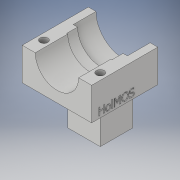
# Autodesk Inventor part: 5.1 Objektivhalterung_Unten
Saved by Autodesk Inventor 2018.3 (Build 223284000, 284)
## iProperties
Part Number: 5.1 Objektivhalterung_Unten
Material: Generisch
Document SubType Name: Modeling
Designer: pgmadmin
Density: 1 g/cm^3
Appearance: Vorgabe
Author: pgmadmin
Autodesk Inventor part; units mm, degrees
ref_plane "YZ Plane" through (0, 0, 0) normal (1, 0, 0) x (0, 1, 0)
ref_plane "XZ Plane" through (0, 0, 0) normal (0, 1, 0) x (-1, 0, 0)
ref_plane "XY Plane" through (0, 0, 0) normal (0, 0, 1) x (1, 0, 0)
sketch "Skizze1" plane through (0, 0, 0) normal (0, 0, 1) x (1, 0, 0)
  line L0 (-16, 20) -> (16, 20)
  line L1 (16, 20) -> (16, -20)
  line L2 (16, -20) -> (-16, -20)
  line L3 (-16, -20) -> (-16, 20)
  line L4 (-16, 20) -> (16, -20) construction
  line L5 (16, 20) -> (-16, -20) construction
  point P0 (0, 0)
  dimension "d0" = 32
  dimension "d1" = 40
  constraints: 12 end point, 2 midpoint, 2 parallel, 1 horizontal, 1 perpendicular
  measures "d0" distance of L1.end L2.end
  measures "d1" distance of L0.end L1.end
extrude "Extrusion1" add sketch "Skizze1" along normal blind 15
sketch "Skizze2" plane through (-16, -20, 0) normal (0, -1, 0) x (1, 0, 0)
  line L0 (0, 15) -> (32, 15) projected
  line L1 (0, 0) -> (0, 15) projected
  line L2 (32, 0) -> (0, 0) projected
  line L3 (32, 0) -> (32, 15) projected
  line L4 (32, 15) -> (0, 15) projected
  circle A0 centre (16, 15) radius 10
  point P0 (16, 0)
  dimension "d4" = 20
  constraints: 1 centre point, 1 midpoint
  measures "d4" diameter of A0
extrude "Extrusion2" cut sketch "Skizze2" against normal blind 15 contours A0 L0 | L0 A0
sketch "Skizze3" plane through (-16, -5, 0) normal (0, -1, 0) x (1, 0, 0)
  line L0 (0, 0) -> (0, 15) projected
  line L1 (32, 0) -> (0, 0) projected
  line L2 (32, 0) -> (32, 15) projected
  line L3 (26, 15) -> (32, 15) projected
  line L4 (0, 15) -> (6, 15) projected
  line L5 (6, 15) -> (26, 15) projected
  circle A0 centre (16, 15) radius 10.5
  point P0 (16, 0)
  dimension "d7" = 21
  constraints: 1 centre point, 1 midpoint
  measures "d7" diameter of A0
extrude "Extrusion3" cut sketch "Skizze3" against normal blind 5 contours A0 L3 L5 L4 | L4 L5 L3 A0
sketch "Skizze4" plane through (-16, 0, 0) normal (0, -1, 0) x (1, 0, 0)
  line L0 (5.5, 15) -> (26.5, 15) projected
  circle A0 centre (16, 15) radius 12.5
  point P0 (16, 0)
  dimension "d10" = 25
  constraints: 1 centre point, 1 midpoint
  measures "d10" diameter of A0
extrude "Extrusion4" cut sketch "Skizze4" against normal through all
sketch "Skizze5" plane through (0, 0, 15) normal (0, 0, 1) x (1, 0, 0)
  line L0 (-16, 20) -> (-16, -20) projected
  line L1 (-16, -20) -> (-10, -20) projected
  line L2 (-10, -20) -> (-10, -5) projected
  line L3 (10, -5) -> (10, -20) projected
  line L4 (10, -20) -> (16, -20) projected
  line L5 (16, -20) -> (16, 20) projected
  circle A0 centre (-13, -13) radius 1.8
  circle A1 centre (13, -13) radius 1.8
  point P0 (0, 0)
  dimension "d13" = 3.6
  dimension "d14" = 3.6
  dimension "d15" = 7
  dimension "d16" = 7
  dimension "d17" = 3
  dimension "d18" = 3
  constraints: 2 centre point
  measures "d13" diameter of A0
  measures "d14" diameter of A1
  measures "d15" distance from line of L1 A0.centre
  measures "d16" distance from line of L4 A1.centre
  measures "d17" distance from line of L5 A1.centre
  measures "d18" distance from line of L0 A0.centre
extrude "Extrusion5" cut sketch "Skizze5" against normal through all
sketch "Skizze6" plane through (0, 0, 0) normal (0, 0, -1) x (-1, 0, 0)
  line L0 (-7.5, 7.5) -> (7.5, 7.5)
  line L1 (7.5, 7.5) -> (7.5, -7.5)
  line L2 (7.5, -7.5) -> (-7.5, -7.5)
  line L3 (-7.5, -7.5) -> (-7.5, 7.5)
  line L4 (-7.5, 7.5) -> (7.5, -7.5) construction
  line L5 (7.5, 7.5) -> (-7.5, -7.5) construction
  point P0 (0, 0)
  dimension "d21" = 15
  dimension "d22" = 15
  constraints: 12 end point, 2 midpoint, 2 parallel, 1 horizontal, 1 perpendicular
  measures "d21" distance of L1.end L2.end
  measures "d22" distance of L0.end L1.end
extrude "Extrusion6" add sketch "Skizze6" along normal blind 20
sketch "Skizze7" plane through (0, 0, -20) normal (0, 0, -1) x (-1, 0, 0)
  circle A0 centre (0, 0) radius 2.5
  dimension "d25" = 5
  constraints: 1 centre point, 1 coincident
  measures "d25" diameter of A0
extrude "Extrusion7" cut sketch "Skizze7" against normal blind 7
sketch "Skizze8" plane through (0, 0, 0) normal (0, 0, -1) x (-1, 0, 0)
  line L0 (12.5, 20) -> (16, 20) projected
  line L1 (16, 20) -> (16, 10.5)
  line L2 (16, 20) -> (16, -20) projected
  line L3 (16, 10.5) -> (-16, 10.5)
  line L4 (-16, 20) -> (-16, -20) projected
  line L5 (16, 20) -> (-16, 20) projected
  line L6 (-16, 20) -> (16, 20)
  point P0 (0, 0)
  dimension "d28" = 9.5
  constraints: 6 end point, 2 point on line, 1 collinear, 1 perpendicular
  measures "d28" distance of L0.end L1.end
extrude "Extrusion8" cut sketch "Skizze8" along normal mid plane 58.75
sketch "Skizze9" plane through (16, -20, 15) normal (1, 0, 0) x (0, 0, -1)
  line L0 (15, 0) -> (0, 0) projected
  line L1 (14, 0) -> (14, 30.5)
  line L2 (0, 30.5) -> (15, 30.5) projected
  line L3 (15, 30.5) -> (15, 0) projected
  line L4 (14, 5.9024) -> (14, 5.4372)
  line L5 (14, 5.4372) -> (12.2869, 5.4372)
  line L6 (12.2869, 5.4372) -> (12.2869, 3.8262)
  line L7 (12.2869, 3.8262) -> (14, 3.8262)
  line L8 (14, 3.8262) -> (14, 3.361)
  line L9 (14, 3.361) -> (10.5, 3.361)
  line L10 (10.5, 3.361) -> (10.5, 3.8262)
  line L11 (10.5, 3.8262) -> (11.8728, 3.8262)
  line L12 (11.8728, 3.8262) -> (11.8728, 5.4372)
  line L13 (11.8728, 5.4372) -> (10.5, 5.4372)
  line L14 (10.5, 5.4372) -> (10.5, 5.9024)
  line L15 (10.5, 5.9024) -> (14, 5.9024)
  spline S0 degree 2 poles (12.6868, 8.7358) (13.3505, 8.7358) (14.0737, 8.0976) (14.0737, 7.5644) knots 0 0 0 1 2 2 2
  spline S1 degree 2 poles (14.0737, 7.5644) (14.0737, 7.017) (13.3278, 6.3902) (12.6868, 6.3902) knots 0 0 0 1 2 2 2
  spline S2 degree 2 poles (12.6868, 6.3902) (12.0288, 6.3902) (11.2998, 7.0369) (11.2998, 7.5644) knots 0 0 0 1 2 2 2
  spline S3 degree 2 poles (11.2998, 7.5644) (11.2998, 8.0976) (12.0259, 8.7358) (12.6868, 8.7358) knots 0 0 0 1 2 2 2
  spline S4 degree 2 poles (12.6868, 8.2792) (12.1763, 8.2792) (11.6799, 7.9076) (11.6799, 7.5644) knots 0 0 0 1 2 2 2
  spline S5 degree 2 poles (11.6799, 7.5644) (11.6799, 7.2212) (12.1763, 6.8468) (12.6868, 6.8468) knots 0 0 0 1 2 2 2
  spline S6 degree 2 poles (12.6868, 6.8468) (13.1831, 6.8468) (13.6937, 7.2212) (13.6937, 7.5644) knots 0 0 0 1 2 2 2
  spline S7 degree 2 poles (13.6937, 7.5644) (13.6937, 7.9048) (13.1917, 8.2792) (12.6868, 8.2792) knots 0 0 0 1 2 2 2
  line L16 (14, 9.6406) -> (14, 9.1981)
  line L17 (14, 9.1981) -> (10.344, 9.1981)
  line L18 (10.344, 9.1981) -> (10.344, 9.6406)
  line L19 (10.344, 9.6406) -> (14, 9.6406)
  line L20 (14, 13.325) -> (14, 12.8598)
  line L21 (14, 12.8598) -> (10.985, 12.8598)
  line L22 (10.985, 12.8598) -> (13.0357, 11.9465)
  line L23 (13.0357, 11.9465) -> (13.0357, 11.6629)
  line L24 (13.0357, 11.6629) -> (10.985, 10.7581)
  line L25 (10.985, 10.7581) -> (14, 10.7581)
  line L26 (14, 10.7581) -> (14, 10.3241)
  line L27 (14, 10.3241) -> (10.5, 10.3241)
  line L28 (10.5, 10.3241) -> (10.5, 10.9595)
  line L29 (10.5, 10.9595) -> (12.4485, 11.8331)
  line L30 (12.4485, 11.8331) -> (10.5, 12.6783)
  line L31 (10.5, 12.6783) -> (10.5, 13.325)
  line L32 (10.5, 13.325) -> (14, 13.325)
  spline S8 degree 2 poles (10.8999, 16.5101) (11.1325, 16.7087) (11.8132, 16.9299) (12.25, 16.9299) knots 0 0 0 1 2 2 2
  spline S9 degree 2 poles (12.25, 16.9299) (12.6754, 16.9299) (13.3647, 16.7143) (13.5972, 16.5101) knots 0 0 0 1 2 2 2
  spline S10 degree 2 poles (13.5972, 16.5101) (13.8412, 16.2946) (14.0737, 15.7245) (14.0737, 15.3813) knots 0 0 0 1 2 2 2
  spline S11 degree 2 poles (14.0737, 15.3813) (14.0737, 15.0267) (13.8327, 14.4595) (13.5972, 14.2524) knots 0 0 0 1 2 2 2
  spline S12 degree 2 poles (13.5972, 14.2524) (13.3647, 14.0511) (12.6811, 13.8355) (12.25, 13.8355) knots 0 0 0 1 2 2 2
  spline S13 degree 2 poles (12.25, 13.8355) (11.8104, 13.8355) (11.141, 14.0539) (10.8999, 14.2553) knots 0 0 0 1 2 2 2
  spline S14 degree 2 poles (10.8999, 14.2553) (10.6673, 14.4595) (10.4263, 15.0296) (10.4263, 15.3813) knots 0 0 0 1 2 2 2
  spline S15 degree 2 poles (10.4263, 15.3813) (10.4263, 15.7387) (10.6759, 16.3116) (10.8999, 16.5101) knots 0 0 0 1 2 2 2
  spline S16 degree 2 poles (12.25, 16.4449) (11.904, 16.4449) (11.3679, 16.2946) (11.1921, 16.1584) knots 0 0 0 1 2 2 2
  spline S17 degree 2 poles (11.1921, 16.1584) (11.0105, 16.0194) (10.829, 15.628) (10.829, 15.3841) knots 0 0 0 1 2 2 2
  spline S18 degree 2 poles (10.829, 15.3841) (10.829, 15.1317) (11.0049, 14.7516) (11.1921, 14.607) knots 0 0 0 1 2 2 2
  spline S19 degree 2 poles (11.1921, 14.607) (11.3707, 14.468) (11.9096, 14.3205) (12.25, 14.3205) knots 0 0 0 1 2 2 2
  spline S20 degree 2 poles (12.25, 14.3205) (12.9392, 14.3205) (13.671, 14.8991) (13.671, 15.3841) knots 0 0 0 1 2 2 2
  spline S21 degree 2 poles (13.671, 15.3841) (13.671, 15.8691) (12.9392, 16.4449) (12.25, 16.4449) knots 0 0 0 1 2 2 2
  spline S22 degree 2 poles (14.0624, 18.4161) (14.0624, 18.0361) (13.9036, 17.5028) (13.7901, 17.2674) knots 0 0 0 1 2 2 2
  line L33 (13.7901, 17.2674) -> (13.2058, 17.2674)
  line L34 (13.2058, 17.2674) -> (13.2058, 17.3015)
  spline S23 degree 2 poles (13.2058, 17.3015) (13.4214, 17.5312) (13.6596, 18.1126) (13.6596, 18.3821) knots 0 0 0 1 2 2 2
  spline S24 degree 2 poles (13.6596, 18.3821) (13.6596, 18.7678) (13.3391, 19.1621) (13.0754, 19.1621) knots 0 0 0 1 2 2 2
  spline S25 degree 2 poles (13.0754, 19.1621) (12.8655, 19.1621) (12.6045, 18.955) (12.5393, 18.731) knots 0 0 0 1 2 2 2
  spline S26 degree 2 poles (12.5393, 18.731) (12.4939, 18.5693) (12.4315, 18.2998) (12.3805, 18.0985) knots 0 0 0 1 2 2 2
  spline S27 degree 2 poles (12.3805, 18.0985) (12.3323, 17.9169) (12.1876, 17.6305) (12.0713, 17.5199) knots 0 0 0 1 2 2 2
  spline S28 degree 2 poles (12.0713, 17.5199) (11.955, 17.4121) (11.643, 17.293) (11.4388, 17.293) knots 0 0 0 1 2 2 2
  spline S29 degree 2 poles (11.4388, 17.293) (11.0134, 17.293) (10.4376, 17.9566) (10.4376, 18.47) knots 0 0 0 1 2 2 2
  spline S30 degree 2 poles (10.4376, 18.47) (10.4376, 18.765) (10.5539, 19.2869) (10.6645, 19.5109) knots 0 0 0 1 2 2 2
  line L35 (10.6645, 19.5109) -> (11.2204, 19.5109)
  line L36 (11.2204, 19.5109) -> (11.2204, 19.4769)
  spline S31 degree 2 poles (11.2204, 19.4769) (11.0673, 19.3096) (10.8404, 18.7877) (10.8404, 18.5012) knots 0 0 0 1 2 2 2
  spline S32 degree 2 poles (10.8404, 18.5012) (10.8404, 18.1779) (11.1438, 17.778) (11.3906, 17.778) knots 0 0 0 1 2 2 2
  spline S33 degree 2 poles (11.3906, 17.778) (11.6118, 17.778) (11.8756, 18.0134) (11.9352, 18.2346) knots 0 0 0 1 2 2 2
  spline S34 degree 2 poles (11.9352, 18.2346) (11.9749, 18.3821) (12.077, 18.8104) (12.1195, 18.9522) knots 0 0 0 1 2 2 2
  spline S35 degree 2 poles (12.1195, 18.9522) (12.2301, 19.3124) (12.6754, 19.6471) (13.0016, 19.6471) knots 0 0 0 1 2 2 2
  spline S36 degree 2 poles (13.0016, 19.6471) (13.2087, 19.6471) (13.6058, 19.4797) (13.7447, 19.3294) knots 0 0 0 1 2 2 2
  spline S37 degree 2 poles (13.7447, 19.3294) (13.8979, 19.1621) (14.0624, 18.7366) (14.0624, 18.4161) knots 0 0 0 1 2 2 2
  point P0 (15, 20)
  dimension "d31" = 1
  constraints: 2 end point, 2 point on line, 2 vertical
  measures "d31" distance between parallel lines of L1 L3
extrude "Extrusion9" cut sketch "Skizze9" against normal blind 2 contours L9 L10 L11 L12 L13 L14 L15 L1 L5 L6 L7 | S37 S22 L1 | L1 S22 L33 L34 S23 S24 S25 S26 S27 S28 S29 S30 L35 L36 S31 S32 S33 S34 S35 S36 S37 | S10 S11 L1 | L1 S11 S12 S13 S14 S15 S8 S9 S10 | S1 S2 S3 S0 L1 | L1 S0 S1 | L1 L21 L22 L23 L24 L25 L27 L28 L29 L30 L31 L32 | L17 L18 L19 L1
sketch "Skizze10" plane through (-16, -20, 0) normal (-1, 0, 0) x (0, 0, 1)
  line L0 (1, 30.5408) -> (1, 0)
  line L1 (0, 0) -> (15, 0) projected
  line L2 (0, 0) -> (0, 30.5) projected
  line L3 (1, 15.3671) -> (1, 15.8323)
  line L4 (1, 15.8323) -> (2.7131, 15.8323)
  line L5 (2.7131, 15.8323) -> (2.7131, 17.4433)
  line L6 (2.7131, 17.4433) -> (1, 17.4433)
  line L7 (1, 17.4433) -> (1, 17.9084)
  line L8 (1, 17.9084) -> (4.5, 17.9084)
  line L9 (4.5, 17.9084) -> (4.5, 17.4433)
  line L10 (4.5, 17.4433) -> (3.1272, 17.4433)
  line L11 (3.1272, 17.4433) -> (3.1272, 15.8323)
  line L12 (3.1272, 15.8323) -> (4.5, 15.8323)
  line L13 (4.5, 15.8323) -> (4.5, 15.3671)
  line L14 (4.5, 15.3671) -> (1, 15.3671)
  spline S0 degree 2 poles (2.3132, 12.5336) (1.6495, 12.5336) (0.9263, 13.1718) (0.9263, 13.705) knots 0 0 0 1 2 2 2
  spline S1 degree 2 poles (0.9263, 13.705) (0.9263, 14.2524) (1.6722, 14.8793) (2.3132, 14.8793) knots 0 0 0 1 2 2 2
  spline S2 degree 2 poles (2.3132, 14.8793) (2.9712, 14.8793) (3.7002, 14.2326) (3.7002, 13.705) knots 0 0 0 1 2 2 2
  spline S3 degree 2 poles (3.7002, 13.705) (3.7002, 13.1718) (2.9741, 12.5336) (2.3132, 12.5336) knots 0 0 0 1 2 2 2
  spline S4 degree 2 poles (2.3132, 12.9903) (2.8237, 12.9903) (3.3201, 13.3618) (3.3201, 13.705) knots 0 0 0 1 2 2 2
  spline S5 degree 2 poles (3.3201, 13.705) (3.3201, 14.0482) (2.8237, 14.4226) (2.3132, 14.4226) knots 0 0 0 1 2 2 2
  spline S6 degree 2 poles (2.3132, 14.4226) (1.8169, 14.4226) (1.3063, 14.0482) (1.3063, 13.705) knots 0 0 0 1 2 2 2
  spline S7 degree 2 poles (1.3063, 13.705) (1.3063, 13.3647) (1.8083, 12.9903) (2.3132, 12.9903) knots 0 0 0 1 2 2 2
  line L15 (1, 11.6289) -> (1, 12.0713)
  line L16 (1, 12.0713) -> (4.656, 12.0713)
  line L17 (4.656, 12.0713) -> (4.656, 11.6289)
  line L18 (4.656, 11.6289) -> (1, 11.6289)
  line L19 (1, 7.9445) -> (1, 8.4096)
  line L20 (1, 8.4096) -> (4.015, 8.4096)
  line L21 (4.015, 8.4096) -> (1.9643, 9.3229)
  line L22 (1.9643, 9.3229) -> (1.9643, 9.6066)
  line L23 (1.9643, 9.6066) -> (4.015, 10.5113)
  line L24 (4.015, 10.5113) -> (1, 10.5113)
  line L25 (1, 10.5113) -> (1, 10.9453)
  line L26 (1, 10.9453) -> (4.5, 10.9453)
  line L27 (4.5, 10.9453) -> (4.5, 10.31)
  line L28 (4.5, 10.31) -> (2.5515, 9.4364)
  line L29 (2.5515, 9.4364) -> (4.5, 8.5912)
  line L30 (4.5, 8.5912) -> (4.5, 7.9445)
  line L31 (4.5, 7.9445) -> (1, 7.9445)
  spline S8 degree 2 poles (4.1001, 4.7593) (3.8675, 4.5608) (3.1868, 4.3395) (2.75, 4.3395) knots 0 0 0 1 2 2 2
  spline S9 degree 2 poles (2.75, 4.3395) (2.3246, 4.3395) (1.6353, 4.5551) (1.4028, 4.7593) knots 0 0 0 1 2 2 2
  spline S10 degree 2 poles (1.4028, 4.7593) (1.1588, 4.9749) (0.9263, 5.545) (0.9263, 5.8882) knots 0 0 0 1 2 2 2
  spline S11 degree 2 poles (0.9263, 5.8882) (0.9263, 6.2427) (1.1673, 6.81) (1.4028, 7.017) knots 0 0 0 1 2 2 2
  spline S12 degree 2 poles (1.4028, 7.017) (1.6353, 7.2184) (2.3189, 7.434) (2.75, 7.434) knots 0 0 0 1 2 2 2
  spline S13 degree 2 poles (2.75, 7.434) (3.1896, 7.434) (3.859, 7.2156) (4.1001, 7.0142) knots 0 0 0 1 2 2 2
  spline S14 degree 2 poles (4.1001, 7.0142) (4.3327, 6.81) (4.5737, 6.2399) (4.5737, 5.8882) knots 0 0 0 1 2 2 2
  spline S15 degree 2 poles (4.5737, 5.8882) (4.5737, 5.5308) (4.3241, 4.9579) (4.1001, 4.7593) knots 0 0 0 1 2 2 2
  spline S16 degree 2 poles (2.75, 4.8246) (3.096, 4.8246) (3.6321, 4.9749) (3.8079, 5.111) knots 0 0 0 1 2 2 2
  spline S17 degree 2 poles (3.8079, 5.111) (3.9895, 5.25) (4.171, 5.6414) (4.171, 5.8853) knots 0 0 0 1 2 2 2
  spline S18 degree 2 poles (4.171, 5.8853) (4.171, 6.1378) (3.9951, 6.5178) (3.8079, 6.6625) knots 0 0 0 1 2 2 2
  spline S19 degree 2 poles (3.8079, 6.6625) (3.6293, 6.8015) (3.0904, 6.9489) (2.75, 6.9489) knots 0 0 0 1 2 2 2
  spline S20 degree 2 poles (2.75, 6.9489) (2.0608, 6.9489) (1.329, 6.3703) (1.329, 5.8853) knots 0 0 0 1 2 2 2
  spline S21 degree 2 poles (1.329, 5.8853) (1.329, 5.4003) (2.0608, 4.8246) (2.75, 4.8246) knots 0 0 0 1 2 2 2
  spline S22 degree 2 poles (0.9376, 2.8533) (0.9376, 3.2334) (1.0964, 3.7666) (1.2099, 4.002) knots 0 0 0 1 2 2 2
  line L32 (1.2099, 4.002) -> (1.7942, 4.002)
  line L33 (1.7942, 4.002) -> (1.7942, 3.968)
  spline S23 degree 2 poles (1.7942, 3.968) (1.5786, 3.7383) (1.3404, 3.1568) (1.3404, 2.8874) knots 0 0 0 1 2 2 2
  spline S24 degree 2 poles (1.3404, 2.8874) (1.3404, 2.5016) (1.6609, 2.1074) (1.9246, 2.1074) knots 0 0 0 1 2 2 2
  spline S25 degree 2 poles (1.9246, 2.1074) (2.1345, 2.1074) (2.3955, 2.3144) (2.4607, 2.5385) knots 0 0 0 1 2 2 2
  spline S26 degree 2 poles (2.4607, 2.5385) (2.5061, 2.7002) (2.5685, 2.9696) (2.6195, 3.171) knots 0 0 0 1 2 2 2
  spline S27 degree 2 poles (2.6195, 3.171) (2.6677, 3.3525) (2.8124, 3.639) (2.9287, 3.7496) knots 0 0 0 1 2 2 2
  spline S28 degree 2 poles (2.9287, 3.7496) (3.045, 3.8574) (3.357, 3.9765) (3.5612, 3.9765) knots 0 0 0 1 2 2 2
  spline S29 degree 2 poles (3.5612, 3.9765) (3.9866, 3.9765) (4.5624, 3.3128) (4.5624, 2.7994) knots 0 0 0 1 2 2 2
  spline S30 degree 2 poles (4.5624, 2.7994) (4.5624, 2.5045) (4.4461, 1.9826) (4.3355, 1.7585) knots 0 0 0 1 2 2 2
  line L34 (4.3355, 1.7585) -> (3.7796, 1.7585)
  line L35 (3.7796, 1.7585) -> (3.7796, 1.7925)
  spline S31 degree 2 poles (3.7796, 1.7925) (3.9327, 1.9599) (4.1596, 2.4818) (4.1596, 2.7682) knots 0 0 0 1 2 2 2
  spline S32 degree 2 poles (4.1596, 2.7682) (4.1596, 3.0916) (3.8562, 3.4915) (3.6094, 3.4915) knots 0 0 0 1 2 2 2
  spline S33 degree 2 poles (3.6094, 3.4915) (3.3882, 3.4915) (3.1244, 3.2561) (3.0648, 3.0348) knots 0 0 0 1 2 2 2
  spline S34 degree 2 poles (3.0648, 3.0348) (3.0251, 2.8874) (2.923, 2.4591) (2.8805, 2.3173) knots 0 0 0 1 2 2 2
  spline S35 degree 2 poles (2.8805, 2.3173) (2.7699, 1.9571) (2.3246, 1.6224) (1.9984, 1.6224) knots 0 0 0 1 2 2 2
  spline S36 degree 2 poles (1.9984, 1.6224) (1.7913, 1.6224) (1.3942, 1.7897) (1.2553, 1.94) knots 0 0 0 1 2 2 2
  spline S37 degree 2 poles (1.2553, 1.94) (1.1021, 2.1074) (0.9376, 2.5328) (0.9376, 2.8533) knots 0 0 0 1 2 2 2
  point P0 (0, 20)
  dimension "d34" = 1
  constraints: 2 end point, 2 vertical, 1 point on line
  measures "d34" distance between parallel lines of L2 L0
extrude "Extrusion10" cut sketch "Skizze10" against normal blind 2 contours L8 L9 L10 L11 L12 L13 L14 L0 L4 L5 L6 | S22 L32 L33 S23 S24 S25 S26 S27 S28 S29 S30 L34 L35 S31 S32 S33 S34 S35 S36 S37 L0 | L0 S37 S22 | S11 S12 S13 S14 S15 S8 S9 S10 L0 | L0 S10 S11 | L26 L27 L28 L29 L30 L31 L0 L20 L21 L22 L23 L24 | L16 L17 L18 L0 | S1 S2 S3 S0 L0 | L0 S0 S1
